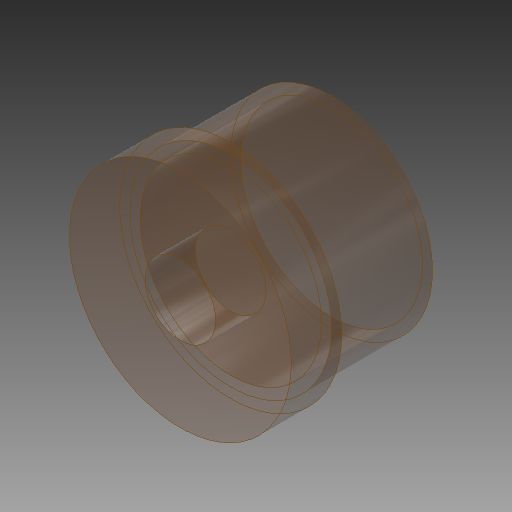
# Autodesk Inventor part: Corpo Valvula Reguladora de Pressão
Saved by Autodesk Inventor 2019 (Build 230136000, 136)
## iProperties
Created: 2020-04-02
Part Number: Corpo Valvula Reguladora de Pressão
Material: Genérico
Document SubType Name: Modeling
Designer: Paulo Rodrigues
Density: 1 g/cm^3
Appearance: Policarbonato - Fumê
Author: Paulo Rodrigues
Autodesk Inventor part; units mm, degrees
ref_plane "YZ Plane" through (0, 0, 0) normal (1, 0, 0) x (0, 1, 0)
ref_plane "XZ Plane" through (0, 0, 0) normal (0, 1, 0) x (-1, 0, 0)
ref_plane "XY Plane" through (0, 0, 0) normal (0, 0, 1) x (1, 0, 0)
sketch "Esboço1" plane through (0, 0, 0) normal (0, 0, 1) x (1, 0, 0)
  circle A0 centre (0, 0) radius 9 projected
  circle A1 centre (0, 0) radius 11
  point P0 (0, 0)
  dimension "d0" = 2
  constraints: 1 centre point
  measures "d0" radial gap between concentric circles of A1 A0
extrude "Extrusão1" add sketch "Esboço1" along normal blind 5 contours A0 | A1
sketch "Esboço2" plane through (0, 0, 0) normal (0, 0, -1) x (-1, 0, 0)
  circle A0 centre (0, 0) radius 9 projected
  circle A1 centre (0, 0) radius 10
  point P0 (0, 0)
  dimension "d3" = 1
  constraints: 1 centre point
  measures "d3" radial gap between concentric circles of A1 A0
extrude "Extrusão2" add sketch "Esboço2" along normal blind 10
hole "Furo1" at (0, 0, 5) direction (0, 0, -1) diameter 7 depth 8 tip angle 118
